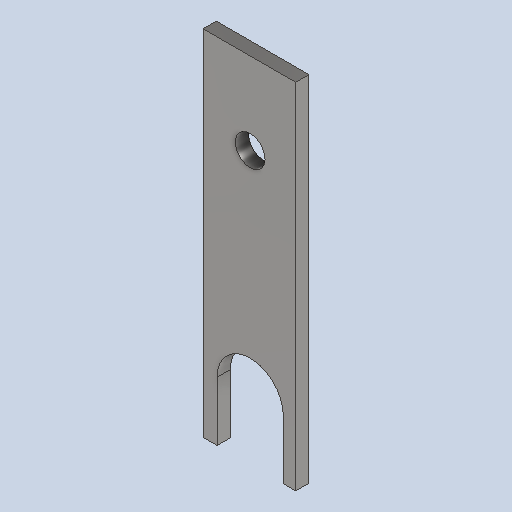
# Autodesk Inventor part: backWheelNoMotor brake mount
Saved by Autodesk Inventor 2022.2 (Build 262287010, 287A)
## iProperties
Created: 2022-04-04
Part Number: backWheelNoMotor brake mount
Material: Steel, Mild
Document SubType Name: Sheet Metal
Designer: foriw
Density: 7.85 g/cm^3
Sheet Metal Rule: Default_mm
Appearance: Semi-Polished
Author: foriw
Autodesk Inventor part; units mm, degrees
ref_plane "YZ Plane" through (0, 0, 0) normal (1, 0, 0) x (0, 1, 0)
ref_plane "XZ Plane" through (0, 0, 0) normal (0, 1, 0) x (-1, 0, 0)
ref_plane "XY Plane" through (0, 0, 0) normal (0, 0, 1) x (1, 0, 0)
sketch "Sketch1" plane through (0, 0, 0) normal (0, 0, 1) x (1, 0, 0)
  line L0 (0, 33.4599) -> (-14, 33.4599) projected
  line L1 (0, 0) -> (-1.8781, 0) projected
  line L2 (0, 0) -> (-14, 0)
  line L3 (-14, 0) -> (-14, 33.4599)
  line L4 (-14, 33.4599) -> (0, 33.4599)
  line L5 (0, 33.4599) -> (0, 0)
  line L6 (-14, 33.4599) -> (0, 33.4599)
  line L7 (0, 33.4599) -> (0, 53.4599)
  line L8 (0, 53.4599) -> (-14, 53.4599)
  line L9 (-14, 53.4599) -> (-14, 33.4599)
  dimension "d0" = 20
  constraints: 16 end point, 4 parallel, 2 horizontal, 2 perpendicular, 1 point on line
  measures "d0" distance of L7.end L6.end
extrude "Extrusion1" add sketch "Sketch1" along normal blind 2
sketch "Sketch2" plane through (0, 0, 2) normal (0, 0, 1) x (1, 0, 0)
  circle A0 centre (-5.7096, 41.0602) radius 6.15 projected
  circle A1 centre (-5.7096, 41.0602) radius 2.15 projected
  circle A2 centre (-6.8781, 8.9314) radius 17.5 projected
  circle A3 centre (-6.8781, 8.9314) radius 5 projected
  circle A4 centre (-6.8781, 8.9314) radius 32.15
  circle A5 centre (-6.8781, 41.0814) radius 2.25
  line L0 (-6.8781, 8.9314) -> (-6.8781, 22.243) construction
  line L1 (-6.8781, 41.0814) -> (-6.8781, 8.9314) construction
  line L2 (-11.8781, -0.9531) -> (-11.8781, 14.8638)
  line L3 (-11.8781, 14.8638) -> (-1.8781, 14.8638)
  line L4 (-1.8781, 14.8638) -> (-1.8781, -0.9531)
  line L5 (-1.8781, -0.9531) -> (-11.8781, -0.9531)
  arc A6 (-1.8781, 8.9314) -> (-11.8781, 8.9314) centre (-6.8781, 8.9314) ccw projected
  arc A7 (-1.8781, 8.9314) -> (-11.8781, 8.9314) centre (-6.8781, 8.9314) ccw projected
  point P0 (0, 0)
  point P1 (-1.8781, 8.9314)
  point P2 (-11.8781, 8.9314)
  dimension "d3" = 4.5
  dimension "d4" = 0
  constraints: 12 end point, 2 centre point, 2 point on circle, 2 tangent, 2 vertical, 1 coincident, 1 perpendicular
  measures "d3" diameter of A5
  measures "d4" distance between parallel lines of L1 L0
extrude "Extrusion2" cut sketch "Sketch2" against normal through all contours A5 A1 A4 | A4 A1 A5 | A4 A5 A1 | A1 A5 A4 | A3 | L4 L5 L2 A3 picked at (-8.3259, 41.5639) picked at (-8.3126, 40.543) picked at (-6.3657, 40.4163) picked at (-6.3452, 41.7271)
equation "\"BendRadius\" = Thickness"
equation "\"BendReliefWidth\" = Thickness"
equation "\"BendReliefDepth\" = 0.5 * Thickness"
equation "\"CornerReliefSize\" = 4 * Thickness"
equation "\"MinimumRemnant\" = 2 * Thickness"
equation "\"TransitionRadius\" = BendRadius"
equation "\"JacobiRadiusSize\" = BendRadius"
equation "\"GapSize\" = Thickness"
equation "\"Thickness\" = 2"
body "Solid1"
